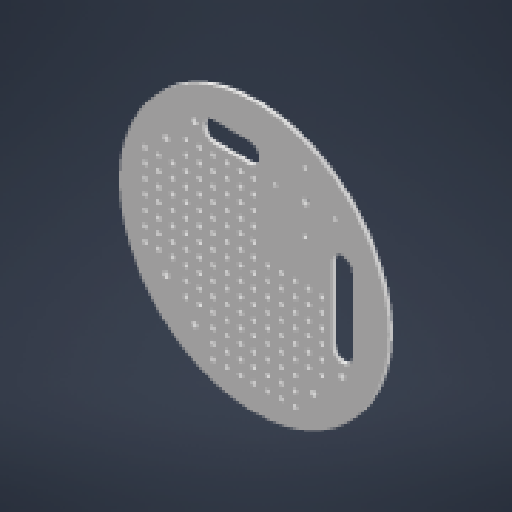
# Autodesk Inventor part: Platform
Saved by Autodesk Inventor 2026.1 (Build 301233020, 233B)
## iProperties
Created: 2026-03-09
Part Number: Platform
Material: Generic
Document SubType Name: Modeling
Designer: Mikke
Density: 1 g/cm^3
Appearance: Default
Author: Mikke
Autodesk Inventor part; units mm, degrees
ref_plane "YZ Plane" through (0, 0, 0) normal (1, 0, 0) x (0, 1, 0)
ref_plane "XZ Plane" through (0, 0, 0) normal (0, 1, 0) x (-1, 0, 0)
ref_plane "XY Plane" through (0, 0, 0) normal (0, 0, 1) x (1, 0, 0)
sketch "Sketch2" plane through (0, 0, 0) normal (0, 0, 1) x (1, 0, 0)
  arc A0 (-15.7199, 60.6781) -> (-34.0297, 78.9878) centre (-90.4651, 4.2426) ccw projected
  line L0 (-14.6737, 61.0337) -> (-15.7199, 60.6781) projected
  arc A1 (-8.1943, -42.6729) -> (-14.6737, 61.0337) centre (-90.4651, 4.2426) ccw projected
  line L1 (-8.1943, -42.6729) -> (-20.7966, -30.0705) projected
  arc A2 (-20.7966, -30.0705) -> (-27.8677, -30.0705) centre (-24.3322, -33.606) ccw projected
  line L2 (-27.8677, -30.0705) -> (-56.152, -58.3548) projected
  arc A3 (-56.152, -58.3548) -> (-56.152, -65.4258) centre (-52.6165, -61.8903) ccw projected
  line L3 (-56.152, -65.4258) -> (-43.5496, -78.0282) projected
  arc A4 (-137.3806, -78.0282) -> (-43.5496, -78.0282) centre (-90.4651, 4.2426) ccw projected
  line L4 (-137.3806, -78.0282) -> (-124.7782, -65.4258) projected
  arc A5 (-124.7782, -65.4258) -> (-124.7782, -58.3548) centre (-128.3138, -61.8903) ccw projected
  line L5 (-124.7782, -58.3548) -> (-153.0625, -30.0705) projected
  arc A6 (-153.0625, -30.0705) -> (-160.1336, -30.0705) centre (-156.598, -33.606) ccw projected
  line L6 (-160.1336, -30.0705) -> (-172.736, -42.6729) projected
  arc A7 (-172.736, 51.1582) -> (-172.736, -42.6729) centre (-90.4651, 4.2426) ccw projected
  line L7 (-172.736, 51.1582) -> (-160.1336, 38.5558) projected
  arc A8 (-160.1336, 38.5558) -> (-153.0625, 38.5558) centre (-156.598, 42.0913) ccw projected
  line L8 (-153.0625, 38.5558) -> (-124.7782, 66.84) projected
  arc A9 (-124.7782, 66.84) -> (-124.7782, 73.9111) centre (-128.3138, 70.3756) ccw projected
  line L9 (-124.7782, 73.9111) -> (-137.3806, 86.5135) projected
  arc A10 (-33.674, 80.034) -> (-137.3806, 86.5135) centre (-90.4651, 4.2426) ccw projected
  line L10 (-34.0297, 78.9878) -> (-33.674, 80.034) projected
  circle A11 centre (-90.4651, 4.2426) radius 98.723 projected
  circle A12 centre (-133.9706, -60.4761) radius 2.25 projected
  circle A13 centre (-155.1838, -39.2629) radius 2.25 projected
  circle A14 centre (-155.1838, 47.7482) radius 2.25 projected
  circle A15 centre (-133.9706, 68.9614) radius 2.25 projected
  circle A16 centre (-46.9596, -60.4761) radius 2.25 projected
  circle A17 centre (-25.7464, -39.2629) radius 2.25 projected
  circle A18 centre (-52.9194, 36.1773) radius 1.5 projected
  circle A19 centre (-30.999, 58.0977) radius 1.5 projected
  circle A20 centre (-52.9194, 58.0977) radius 2.5 projected
  circle A21 centre (-74.8397, 58.0977) radius 1.5 projected
  circle A22 centre (-52.9194, 80.018) radius 1.5 projected
  circle A23 centre (-90.4651, 4.2426) radius 98.723
  point P0 (0, 0)
  constraints: 1 centre point, 1 coincident, 1 concentric
extrude "Extrusion2" add sketch "Sketch2" along normal blind 3 contours L0 A1 L1 A2 L2 A3 L3 A4 L4 A5 L5 A6 L6 A7 L7 A8 L8 A9 L9 A10 L10 A0 | A11
sketch "Sketch3" plane through (-90.4651, 4.2426, 3) normal (0, 0, 1) x (1, 0, 0)
  line L0 (-50, 0) -> (-50, -50)
  line L1 (-50, -50) -> (0, -50)
  circle A0 centre (-50, -50) radius 1.75
  point P0 (90.4651, -4.2426)
  dimension "d6" = 50
  dimension "d7" = 50
  dimension "d8" = 3.5
  constraints: 4 end point, 1 centre point, 1 coincident
  measures "d6" distance of L1.end L0.end
  measures "d7" distance of L0.end L0.start
  measures "d8" diameter of A0
extrude "Extrusion3" cut sketch "Sketch3" against normal blind 3
pattern_linear "Rectangular Pattern1" count 11 spacing 10 along (0, 1, 0) count 6 spacing 10 along (1, 0, 0) of "Extrusion3"
pattern_linear "Rectangular Pattern2" count 6 spacing 10 along (0, 1, 0) count 11 spacing 10 along (1, 0, 0) of "Extrusion3"
sketch "Sketch4" plane through (-90.4651, 4.2426, 3) normal (0, 0, 1) x (1, 0, 0)
  circle A0 centre (-30, -50) radius 1.75 projected
  line L0 (-30, -50) -> (-30, -60)
  line L1 (-30, -50) -> (-20, -50) construction
  line L2 (-30, -60) -> (-30, -70)
  line L3 (-30, -70) -> (-30, -80)
  circle A1 centre (-30, -80) radius 1.75
  point P0 (90.4651, -4.2426)
  dimension "d23" = 10
  dimension "d24" = 90
  dimension "d28" = 10
  dimension "d29" = 10
  dimension "d30" = 3.5
  constraints: 8 end point, 2 coincident, 2 vertical, 1 centre point, 1 horizontal, 1 perpendicular, 1 point on line
  measures "d23" distance of L0.start L0.end
  measures "d24" angle of L0 L1
  measures "d28" distance of L2.start L2.end
  measures "d29" distance of L2.end L3.end
  measures "d30" diameter of A1
extrude "Extrusion4" cut sketch "Sketch4" against normal blind 3 contours A1
pattern_linear "Rectangular Pattern3" count 3 spacing 10 along (0, 1, 0) count 7 spacing 10 along (1, 0, 0) of "Extrusion4"
sketch "Sketch5" plane through (-90.4651, 4.2426, 3) normal (0, 0, 1) x (1, 0, 0)
  circle A0 centre (-50, -30) radius 1.75 projected
  line L0 (-50, -30) -> (-80, -30)
  circle A1 centre (-80, -30) radius 1.75
  point P0 (90.4651, -4.2426)
  dimension "d37" = 30
  dimension "d38" = 3.5
  constraints: 2 end point, 1 centre point, 1 coincident, 1 horizontal
  measures "d37" distance of L0.start L0.end
  measures "d38" diameter of A1
extrude "Extrusion5" cut sketch "Sketch5" against normal blind 3 contours A1
pattern_linear "Rectangular Pattern4" count 7 spacing 10 along (0, 1, 0) count 3 spacing 10 along (1, 0, 0) of "Extrusion5"
sketch "Sketch6" plane through (-90.4651, 4.2426, 3) normal (0, 0, 1) x (1, 0, 0)
  circle A0 centre (-60, 30) radius 1.75 construction
  circle A1 centre (-60, 20) radius 1.75 construction
  circle A2 centre (-60, 10) radius 1.75 construction
  circle A3 centre (-60, 0) radius 1.75 construction
  circle A4 centre (-60, -10) radius 1.75 construction
  circle A5 centre (-60, -20) radius 1.75 construction
  circle A6 centre (-60, -30) radius 1.75 construction
  circle A7 centre (-70, 30) radius 1.75 construction
  circle A8 centre (-70, 20) radius 1.75 construction
  circle A9 centre (-70, 10) radius 1.75 construction
  circle A10 centre (-70, 0) radius 1.75 construction
  circle A11 centre (-70, -10) radius 1.75 construction
  circle A12 centre (-70, -20) radius 1.75 construction
  circle A13 centre (-70, -30) radius 1.75 construction
  circle A14 centre (-80, 30) radius 1.75 construction
  circle A15 centre (-80, 20) radius 1.75 construction
  circle A16 centre (-80, 10) radius 1.75 construction
  circle A17 centre (-80, 0) radius 1.75 construction
  circle A18 centre (-80, -10) radius 1.75 construction
  circle A19 centre (-80, -20) radius 1.75 construction
  circle A20 centre (-80, -30) radius 1.75 construction
  circle A21 centre (30, -60) radius 1.75 construction
  circle A22 centre (30, -70) radius 1.75 construction
  circle A23 centre (30, -80) radius 1.75 construction
  circle A24 centre (20, -60) radius 1.75 construction
  circle A25 centre (20, -70) radius 1.75 construction
  circle A26 centre (20, -80) radius 1.75 construction
  circle A27 centre (10, -60) radius 1.75 construction
  circle A28 centre (10, -70) radius 1.75 construction
  circle A29 centre (10, -80) radius 1.75 construction
  circle A30 centre (0, -60) radius 1.75 construction
  circle A31 centre (0, -70) radius 1.75 construction
  circle A32 centre (0, -80) radius 1.75 construction
  circle A33 centre (-10, -60) radius 1.75 construction
  circle A34 centre (-10, -70) radius 1.75 construction
  circle A35 centre (-10, -80) radius 1.75 construction
  circle A36 centre (-20, -60) radius 1.75 construction
  circle A37 centre (-20, -70) radius 1.75 construction
  circle A38 centre (-20, -80) radius 1.75 construction
  circle A39 centre (-30, -60) radius 1.75 construction
  circle A40 centre (-30, -70) radius 1.75 construction
  circle A41 centre (-30, -80) radius 1.75 construction
  circle A42 centre (50, 0) radius 1.75 construction
  circle A43 centre (50, -10) radius 1.75 construction
  circle A44 centre (50, -20) radius 1.75 construction
  circle A45 centre (50, -30) radius 1.75 construction
  circle A46 centre (50, -40) radius 1.75 construction
  circle A47 centre (50, -50) radius 1.75 construction
  circle A48 centre (40, 0) radius 1.75 construction
  circle A49 centre (40, -10) radius 1.75 construction
  circle A50 centre (40, -20) radius 1.75 construction
  circle A51 centre (40, -30) radius 1.75 construction
  circle A52 centre (40, -40) radius 1.75 construction
  circle A53 centre (40, -50) radius 1.75 construction
  circle A54 centre (30, 0) radius 1.75 construction
  circle A55 centre (30, -10) radius 1.75 construction
  circle A56 centre (30, -20) radius 1.75 construction
  circle A57 centre (30, -30) radius 1.75 construction
  circle A58 centre (30, -40) radius 1.75 construction
  circle A59 centre (30, -50) radius 1.75 construction
  circle A60 centre (20, 0) radius 1.75 construction
  circle A61 centre (20, -10) radius 1.75 construction
  circle A62 centre (20, -20) radius 1.75 construction
  circle A63 centre (20, -30) radius 1.75 construction
  circle A64 centre (20, -40) radius 1.75 construction
  circle A65 centre (20, -50) radius 1.75 construction
  circle A66 centre (10, 0) radius 1.75 construction
  circle A67 centre (10, -10) radius 1.75 construction
  circle A68 centre (10, -20) radius 1.75 construction
  circle A69 centre (10, -30) radius 1.75 construction
  circle A70 centre (10, -40) radius 1.75 construction
  circle A71 centre (10, -50) radius 1.75 construction
  circle A72 centre (0, 50) radius 1.75 construction
  circle A73 centre (0, 40) radius 1.75 construction
  circle A74 centre (0, 30) radius 1.75 construction
  circle A75 centre (0, 20) radius 1.75 construction
  circle A76 centre (0, 10) radius 1.75 construction
  circle A77 centre (0, 0) radius 1.75 construction
  circle A78 centre (0, -10) radius 1.75 construction
  circle A79 centre (0, -20) radius 1.75 construction
  circle A80 centre (0, -30) radius 1.75 construction
  circle A81 centre (0, -40) radius 1.75 construction
  circle A82 centre (0, -50) radius 1.75 construction
  circle A83 centre (-10, 50) radius 1.75 construction
  circle A84 centre (-10, 40) radius 1.75 construction
  circle A85 centre (-10, 30) radius 1.75 construction
  circle A86 centre (-10, 20) radius 1.75 construction
  circle A87 centre (-10, 10) radius 1.75 construction
  circle A88 centre (-10, 0) radius 1.75 construction
  circle A89 centre (-10, -10) radius 1.75 construction
  circle A90 centre (-10, -20) radius 1.75 construction
  circle A91 centre (-10, -30) radius 1.75 construction
  circle A92 centre (-10, -40) radius 1.75 construction
  circle A93 centre (-10, -50) radius 1.75 construction
  circle A94 centre (-20, 50) radius 1.75 construction
  circle A95 centre (-20, 40) radius 1.75 construction
  circle A96 centre (-20, 30) radius 1.75 construction
  circle A97 centre (-20, 20) radius 1.75 construction
  circle A98 centre (-20, 10) radius 1.75 construction
  circle A99 centre (-20, 0) radius 1.75 construction
  circle A100 centre (-20, -10) radius 1.75 construction
  circle A101 centre (-20, -20) radius 1.75 construction
  circle A102 centre (-20, -30) radius 1.75 construction
  circle A103 centre (-20, -40) radius 1.75 construction
  circle A104 centre (-20, -50) radius 1.75 construction
  circle A105 centre (-30, 50) radius 1.75 construction
  circle A106 centre (-30, 40) radius 1.75 construction
  circle A107 centre (-30, 30) radius 1.75 construction
  circle A108 centre (-30, 20) radius 1.75 construction
  circle A109 centre (-30, 10) radius 1.75 construction
  circle A110 centre (-30, 0) radius 1.75 construction
  circle A111 centre (-30, -10) radius 1.75 construction
  circle A112 centre (-30, -20) radius 1.75 construction
  circle A113 centre (-30, -30) radius 1.75 construction
  circle A114 centre (-30, -40) radius 1.75 construction
  circle A115 centre (-30, -50) radius 1.75 construction
  circle A116 centre (-40, 50) radius 1.75 construction
  circle A117 centre (-40, 40) radius 1.75 construction
  circle A118 centre (-40, 30) radius 1.75 construction
  circle A119 centre (-40, 20) radius 1.75 construction
  circle A120 centre (-40, 10) radius 1.75 construction
  circle A121 centre (-40, 0) radius 1.75 construction
  circle A122 centre (-40, -10) radius 1.75 construction
  circle A123 centre (-40, -20) radius 1.75 construction
  circle A124 centre (-40, -30) radius 1.75 construction
  circle A125 centre (-40, -40) radius 1.75 construction
  circle A126 centre (-40, -50) radius 1.75 construction
  circle A127 centre (-50, 50) radius 1.75 construction
  circle A128 centre (-50, 40) radius 1.75 construction
  circle A129 centre (-50, 30) radius 1.75 construction
  circle A130 centre (-50, 20) radius 1.75 construction
  circle A131 centre (-50, 10) radius 1.75 construction
  circle A132 centre (-50, 0) radius 1.75 construction
  circle A133 centre (-50, -10) radius 1.75 construction
  circle A134 centre (-50, -20) radius 1.75 construction
  circle A135 centre (-50, -30) radius 1.75 construction
  circle A136 centre (-50, -40) radius 1.75 construction
  circle A137 centre (-50, -50) radius 1.75 construction
  circle A138 centre (0, 0) radius 98.723 construction
  circle A139 centre (-43.5055, -64.7187) radius 2.25 construction
  circle A140 centre (-64.7187, -43.5055) radius 2.25 construction
  circle A141 centre (-64.7187, 43.5055) radius 2.25 construction
  circle A142 centre (-43.5055, 64.7187) radius 2.25 construction
  circle A143 centre (43.5055, -64.7187) radius 2.25 construction
  circle A144 centre (64.7187, -43.5055) radius 2.25 construction
  circle A145 centre (37.5458, 75.7753) radius 1.5 construction
  circle A146 centre (15.6254, 53.855) radius 1.5 construction
  circle A147 centre (37.5458, 53.855) radius 2.5 construction
  circle A148 centre (59.4661, 53.855) radius 1.5 construction
  circle A149 centre (37.5458, 31.9347) radius 1.5 construction
  line L0 (64.7187, -43.5055) -> (64.7187, 41.4945)
  line L1 (64.7187, -43.5055) -> (149.7187, -43.5055) construction
  line L2 (-43.5055, 64.7187) -> (6.4945, 64.7187)
  line L3 (72.2187, 25.9247) -> (57.2187, 25.9247)
  arc A150 (72.2187, 25.9247) -> (57.2187, 25.9247) centre (64.7187, 25.9347) ccw
  line L4 (72.2187, -27.8321) -> (57.2187, -27.8321)
  arc A151 (57.2187, -27.8321) -> (72.2187, -27.8321) centre (64.7187, -27.9214) ccw
  line L5 (72.2187, -27.8321) -> (72.2187, 25.9247)
  line L6 (57.2187, -27.8321) -> (57.2187, 25.9247)
  line L7 (-3.6919, 72.2187) -> (-3.6919, 57.2187)
  line L8 (-30, 72.2187) -> (-30, 57.2187)
  arc A152 (-3.6919, 57.2187) -> (-3.6919, 72.2187) centre (-3.6919, 64.7187) ccw
  arc A153 (-30, 72.2187) -> (-30, 57.2187) centre (-30.066, 64.7187) ccw
  line L9 (-3.6919, 57.2187) -> (-30.1319, 57.2187)
  line L10 (-30, 72.2187) -> (-3.6919, 72.2187)
  point P0 (90.4651, -4.2426)
  point P1 (64.7187, 25.9247)
  point P2 (64.7187, -27.8321)
  point P3 (-3.6919, 64.7187)
  point P4 (-30, 64.7187)
  dimension "d47" = 85
  dimension "d48" = 90
  dimension "d49" = 50
  dimension "d50" = 15
  dimension "d51" = 15
  dimension "d52" = 15
  dimension "d53" = 15
  dimension "d54" = 7.5
  constraints: 22 end point, 10 point on circle, 4 centre point, 4 horizontal, 4 midpoint, 4 point on line, 2 parallel, 2 vertical, 1 perpendicular, 1 tangent
  measures "d47" distance of L0.start L0.end
  measures "d48" angle of L1 L0
  measures "d49" distance of L2.start L2.end
  measures "d50" distance of L3.start L3.end
  measures "d51" distance of L4.start L4.end
  measures "d52" distance of L7.start L7.end
  measures "d53" distance of L8.start L8.end
  measures "d54" radius of A152
extrude "Extrusion6" cut sketch "Sketch6" against normal blind 10
body "Solid2"
